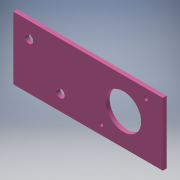
# Autodesk Inventor part: secondaryflywheelmount
Saved by Autodesk Inventor 2016 (Build 200138000, 138)
## iProperties
Created: 2016-02-24
Part Number: secondaryflywheelmount
Material: Generic
Document SubType Name: Modeling
Designer: gus
Density: 1 g/cm^3
Appearance: Pink
Author: gus
Autodesk Inventor part; units mm, degrees
ref_plane "YZ Plane" through (0, 0, 0) normal (1, 0, 0) x (0, 1, 0)
ref_plane "XZ Plane" through (0, 0, 0) normal (0, 1, 0) x (-1, 0, 0)
ref_plane "XY Plane" through (0, 0, 0) normal (0, 0, 1) x (1, 0, 0)
sketch "Sketch1" plane through (0, 0, 0) normal (0, 0, 1) x (1, 0, 0)
  line L0 (0, 0) -> (-120.65, 0)
  line L1 (-120.65, 0) -> (-120.65, -50.8)
  line L2 (-120.65, -50.8) -> (0, -50.8)
  line L3 (0, -50.8) -> (0, 0)
  circle A0 centre (-31.75, -25.4) radius 14.2875
  circle A1 centre (-13.7895, -7.4395) radius 1.5875
  circle A2 centre (-49.7105, -43.3605) radius 1.5875
  dimension "d0" = 28.575
  dimension "d1" = 25.4
  dimension "d2" = 25.4
  dimension "d3" = 50.8
  dimension "d4" = 3.175
  dimension "d5" = 3.175
  dimension "d6" = 25.4
  dimension "d7" = 31.75
  dimension "d8" = 88.9
  dimension "d9" = 17.9605
  dimension "d10" = 17.9605
  constraints: 8 end point, 3 centre point, 2 parallel, 1 horizontal, 1 perpendicular
  measures "d0" diameter of A0
  measures "d1" distance from line of L0 A0.centre
  measures "d2" distance from line of L2 A0.centre
  measures "d3" distance of A2.centre A1.centre
  measures "d4" diameter of A1
  measures "d5" diameter of A2
  measures "d6" distance of A1.centre A0.centre
  measures "d7" distance from line of L3 A0.centre
  measures "d8" distance from line of A0.centre L1
  measures "d9" horizontal distance of A0.centre A1.centre
  measures "d10" horizontal distance of A0.centre A2.centre
extrude "Extrusion1" add sketch "Sketch1" along normal blind 3.175
sketch "Sketch2" plane through (0, 0, 3.175) normal (0, 0, 1) x (1, 0, 0)
  circle A0 centre (-107.95, -12.7) radius 3.3734
  line L0 (-120.65, 0) -> (-120.65, -50.8) projected
  line L1 (0, 0) -> (-120.65, 0) projected
  circle A1 centre (-82.55, -38.1) radius 3.3734
  line L2 (-120.65, -50.8) -> (0, -50.8) projected
  dimension "d13" = 6.7469
  dimension "d14" = 12.7
  dimension "d15" = 12.7
  dimension "d16" = 6.7469
  dimension "d17" = 12.7
  dimension "d18" = 38.1
  constraints: 2 centre point
  measures "d13" diameter of A0
  measures "d14" distance from line of L0 A0.centre
  measures "d15" distance from line of L1 A0.centre
  measures "d16" diameter of A1
  measures "d17" distance from line of L2 A1.centre
  measures "d18" distance from line of L0 A1.centre
extrude "Extrusion2" cut sketch "Sketch2" against normal blind 3.175
body "Solid1"
